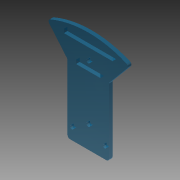
# Autodesk Inventor part: bracket_camera_bottom
Saved by Autodesk Inventor 2015 SP2 (Build 190223200, 223)
## iProperties
Created: 2015-10-08
Part Number: bracket_camera_bottom
Material: Generic
Document SubType Name: Modeling
Designer: styku
Density: 1 g/cm^3
Appearance: Clear
Author: styku
Autodesk Inventor part; units mm, degrees
ref_plane "YZ Plane" through (0, 0, 0) normal (1, 0, 0) x (0, 1, 0)
ref_plane "XZ Plane" through (0, 0, 0) normal (0, 1, 0) x (-1, 0, 0)
ref_plane "XY Plane" through (0, 0, 0) normal (0, 0, 1) x (1, 0, 0)
sketch "Sketch1" plane through (0, 0, 0) normal (0, 1, 0) x (-1, 0, 0)
  line L0 (46, 0) -> (-35, 0) construction
  line L1 (0, 54.3949) -> (0, -60) construction
  line L2 (17, -28) -> (17, 28)
  circle A0 centre (13.5, -18.75) radius 1.5
  line L3 (-17, 28) -> (-17, -28)
  line L4 (17, -28) -> (-17, -28)
  line L5 (17, 28) -> (33.782, 48)
  line L6 (17, 28) -> (43.1081, 28) construction
  line L7 (-17, 28) -> (-33.782, 48)
  arc A1 (33.782, 48) -> (-33.782, 48) centre (0, -24.5174) ccw
  line L8 (20, 48) -> (-20, 48)
  line L9 (-20, 48) -> (-20, 45)
  line L10 (-20, 45) -> (20, 45)
  line L11 (20, 45) -> (20, 48)
  circle A2 centre (0, 35) radius 1.5
  circle A3 centre (-13.5, -18.75) radius 1.5
  circle A4 centre (0, -10) radius 1.625
  line L12 (10, 31) -> (-10, 31)
  line L13 (-10, 31) -> (-10, 28)
  line L14 (-10, 28) -> (10, 28)
  line L15 (10, 28) -> (10, 31)
  point P0 (0, 0)
  dimension "d16" = 3
  dimension "d35" = 50
  dimension "d36" = 20
  dimension "d37" = 56
  dimension "d38" = 80
  dimension "d39" = 40
  dimension "d41" = 3
  dimension "d43" = 9.25
  dimension "d44" = 3
  dimension "d45" = 10
  dimension "d49" = 45
  dimension "d50" = 34
  dimension "d51" = 28
  dimension "d52" = 13.5
  dimension "d53" = 3.25
  dimension "d54" = 18
  dimension "d58" = 20
  dimension "d59" = 28
  dimension "d60" = 3
  constraints: 32 end point, 5 centre point, 5 horizontal, 4 parallel, 4 vertical, 3 perpendicular, 2 equal length, 2 point on circle, 2 point on line, 2 symmetric about line, 4 other
  measures "d16" diameter of A0
  measures "d35" angle of L6 L5
  measures "d36" vertical distance of L3.start L7.end
  measures "d37" distance of L3.start L3.end
  measures "d38" radius of A1
  measures "d39" distance of L8.start L8.end
  measures "d41" distance of L8.end L9.end
  measures "d43" distance from line of L4 A0.centre
  measures "d44" diameter of A2
  measures "d45" distance from line of L10 A2.centre
  measures "d49" distance between parallel lines of L0 L10
  measures "d50" distance between parallel lines of L2 L3
  measures "d51" distance between parallel lines of L4 L0
  measures "d52" distance from line of L1 A3.centre
  measures "d53" diameter of A4
  measures "d54" distance from line of L4 A4.centre
  measures "d58" distance between parallel lines of L13 L15
  measures "d59" distance between parallel lines of L0 L14
  measures "d60" distance of L12.end L13.end
extrude "Extrusion3" add sketch "Sketch1" along normal blind 3 contours L4 L3 L7 A1 L5 L2 | L15 L14 L13 L12
fillet "Fillet3" radius 2 6 edges at (-33.782, 1.5, 48) (-17, 1.5, 28) (33.782, 1.5, 48) (17, 1.5, 28) (-17, 1.5, -28) (17, 1.5, -28)
extrude "Extrusion4" cut sketch "Sketch1" along normal blind 3 contours L15 L14 L13 L12
body "Solid3"
